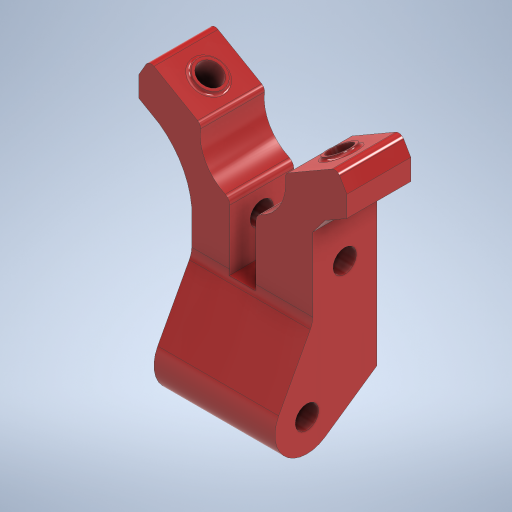
# Autodesk Inventor part: YZ_Roller
Saved by Autodesk Inventor 2023 (Build 270158000, 158)
## iProperties
Created: 2023-11-24
Part Number: YZ_Roller
Material: Generic
Document SubType Name: Modeling
Designer: danie
Density: 1 g/cm^3
Appearance: Default
Author: danie
Autodesk Inventor part; units mm, degrees
ref_plane "YZ Plane" through (0, 0, 0) normal (1, 0, 0) x (0, 1, 0)
ref_plane "XZ Plane" through (0, 0, 0) normal (0, 1, 0) x (-1, 0, 0)
ref_plane "XY Plane" through (0, 0, 0) normal (0, 0, 1) x (1, 0, 0)
sketch "Sketch1" plane through (59.7334, 64.5979, 5.1545) normal (1, 0, 0) x (0, 1, 0)
  line L0 (18.8189, 17.1759) -> (22.8279, 17.1759) projected
  line L1 (18.8189, -4.3241) -> (22.8279, -4.3241) projected
  line L2 (22.3279, -4.8241) -> (19.3338, -4.8241) projected
  arc A0 (-48.3948, 28.867) -> (-62.6447, 12.9256) centre (-53.5949, 19.1757) ccw
  line L3 (-48.3948, 28.867) -> (-28.1429, 18.0072)
  line L4 (-24.8341, 17.1759) -> (22.8279, 17.1759)
  line L5 (22.8279, 17.1759) -> (22.8279, -4.3241)
  line L6 (22.8279, -4.3241) -> (22.8279, -4.8241)
  line L7 (22.8279, -4.8241) -> (22.3279, -4.8241)
  line L8 (22.3279, -4.8241) -> (-50.3885, -4.8241)
  line L9 (-50.3885, -4.8241) -> (-62.6447, 12.9256)
  arc A1 (-28.1429, 18.0072) -> (-24.8341, 17.1759) centre (-24.8333, 24.1792) ccw
  point P0 (-48.3934, 28.8694)
  point P1 (0.4728, 17.1759)
  point P2 (-13.5862, 6.178)
  constraints: 14 end point, 4 point on circle, 2 centre point, 2 perpendicular, 1 coincident, 1 collinear, 1 horizontal, 1 point on line, 1 tangent
sketch "Sketch2" plane through (47.0121, 65.2772, 22.3304) normal (0, 0, 1) x (1, 0, 0)
  line L0 (17.0615, 5.4672) -> (24.4547, 9.7356)
  line L1 (24.4547, 9.7356) -> (24.4547, 16.9356)
  line L2 (24.4547, 16.9356) -> (22.0224, 21.1485)
  arc A0 (22.0224, 21.1485) -> (19.2903, 21.8806) centre (20.2903, 20.1485) ccw
  line L3 (22.0224, 21.1485) -> (20.2903, 20.1485) construction
  line L4 (19.2903, 21.8806) -> (20.2903, 20.1485) construction
  line L5 (19.2903, 21.8806) -> (4.2935, 13.2221)
  arc A1 (4.2935, 13.2221) -> (3.3088, 11.2431) centre (5.2935, 11.4901) ccw
  arc A2 (-25.8662, 11.2431) -> (3.3088, 11.2431) centre (-11.2787, 9.4277) ccw
  arc A3 (-25.8662, 11.2431) -> (-26.8509, 13.2221) centre (-27.8509, 11.4901) ccw
  line L6 (-26.8509, 13.2221) -> (-41.8477, 21.8806)
  arc A4 (-41.8477, 21.8806) -> (-44.5798, 21.1485) centre (-42.8477, 20.1485) ccw
  line L7 (-44.5798, 21.1485) -> (-47.0121, 16.9356)
  line L8 (-47.0121, 16.9356) -> (-47.0121, 16.9356)
  line L9 (-47.0121, 9.7356) -> (-39.9003, 5.6296) projected
  line L10 (-39.926, 5.6445) -> (-39.2899, 5.1683) projected
  line L11 (-39.926, 5.6445) -> (-47.0121, 9.7356)
  arc A5 (-28.8787, -13.5153) -> (-39.926, 5.6445) centre (-55.4557, -16.0746) ccw
  line L12 (12.7213, -0.2066) -> (17.0615, 5.4672)
  line L13 (12.7213, -65.2726) -> (12.7213, -49.0741) projected
  line L14 (12.7213, -65.2726) -> (12.7213, -25.5127)
  line L15 (12.7213, -65.2726) -> (-28.8787, -65.2726)
  line L16 (12.7213, -25.5127) -> (12.7213, -0.2066)
  line L17 (-28.8787, -65.2726) -> (-28.8787, -13.5153)
  line L18 (-47.0121, 9.7356) -> (-47.0121, 16.9356)
  line L19 (-6.7787, -27.2723) -> (-15.7787, -27.2723) projected
  line L20 (-6.7787, -27.2723) -> (-15.7787, -27.2723)
  line L21 (-6.7787, -27.2723) -> (-15.7787, -27.2723)
  line L22 (-15.7787, -27.2723) -> (-15.7787, -3.6713)
  line L23 (-15.7787, -3.6713) -> (-6.7787, -3.6713)
  line L24 (-6.7787, -3.6713) -> (-6.7787, -27.2723)
  arc A6 (-15.7787, -6.4085) -> (-17.3582, -3.9562) centre (-18.4721, -6.4085) ccw
  arc A7 (-5.218, -3.9648) -> (-6.7787, -6.384) centre (-4.1232, -6.384) ccw
  point P0 (-47.0121, -65.2772)
  point P1 (12.7213, -49.0728)
  point P2 (12.7213, -63.3241)
  point P3 (-15.7787, -5.7822)
  dimension "d3" = 2
  dimension "d4" = 90
  dimension "d5" = 2
  dimension "d6" = 26.7
  dimension "d7" = 2
  dimension "d8" = 90
  dimension "d13" = 0
  constraints: 42 end point, 18 point on circle, 8 centre point, 8 tangent, 5 vertical, 3 point on line, 2 collinear, 2 horizontal, 2 parallel, 2 perpendicular
  measures "d3" radius of A0
  measures "d4" angle of L3 L4
  measures "d5" radius of A1
  measures "d6" radius of A5
  measures "d7" radius of A4
  measures "d8" angle of L7 L6
  measures "d13" distance from line of L19.end L22
extrude "Extrusion1" add sketch "Sketch1" along normal mid plane 200
extrude "Extrusion2" cut sketch "Sketch2" along normal mid plane 200 contours L12 L16 L14 L13 L15 L17 A5 L9 L18 L7 A4 L6 A3 A2 A6 L22 L19 L24 A7 A1 L5 A0 L2 L1 L0 keep common part
sketch "Sketch5" plane through (35.7334, 74.705, 22.3304) normal (0, 0, 1) x (1, 0, 0)
  point P0 (-35.7334, -74.705)
sketch "Sketch3" plane through (66.3024, 87.1578, 22.3304) normal (-0.4999998, 0.8660255, 0) x (0.8660255, 0.4999998, 0)
  ellipse E0 centre (-8.9999, 10.9997) end of major axis (-4.913, 11.323) minor radius 4.0997 projected
  point P0 (-100.9985, 22.3304)
  constraints: 1 coincident
sketch "Sketch4" plane through (20.1613, 78.4993, 22.3304) normal (0.5000005, 0.8660251, 0) x (0.8660251, -0.5000005, 0)
  ellipse E0 centre (-8.3172, 10.9997) end of major axis (-5.344, 8.1771) minor radius 4.0996 projected
  point P0 (21.7896, 22.3304)
  constraints: 1 coincident
sketch "Sketch6" plane through (18.1334, 14.2094, 0.3304) normal (-1, 0, 0) x (0, 0, 1)
  point P0 (-0.3304, -14.2094)
hole "Hole1" at (58.5083, 82.6578, 11.3306) direction (0.4999998, -0.8660255, 0) diameter 8 end through all clearance for "Countersunk Flat Head Screw ISO 2009/7046" size "M8" standard "ISO"
hole "Hole2" at (12.9584, 82.6579, 11.3307) direction (-0.5000005, -0.8660251, 0) diameter 8 end through all clearance for "Slotted Cheese Head Screw ISO 1207" size "M8" standard "ISO"
hole "Hole3" at (59.7334, 51.0116, 11.3325) at (59.7334, 11.003, 24.3302) direction (-1, 0, 0) diameter 8 end through all
sketch "Sketch7" plane through (0, 75.0129, 0.3304) normal (-0.4999998, -0.8660255, 0) x (0.8660255, -0.4999998, 0)
  arc A0 (8.1823, 14.923) -> (8.1823, 7.0776) centre (7.3997, 11.0003) ccw projected
  line L0 (8.1823, 14.923) -> (8.1823, 22) projected
  line L1 (8.1823, 22) -> (0, 22) projected
  line L2 (0, 0) -> (0, 22) projected
  line L3 (0, 0) -> (8.1823, 0) projected
  line L4 (8.1823, 0) -> (8.1823, 7.0776) projected
  circle A1 centre (7.3997, 11.0003) radius 7
  point P0 (37.5064, -0.3304)
  dimension "d39" = 14
  constraints: 1 centre point, 1 coincident
  measures "d39" diameter of A1
extrude "Extrusion5" cut sketch "Sketch7" along normal blind 10 contours L0 A1 L4 A0 | A0 L4 A1 L0
sketch "Sketch8" plane through (71.4668, 75.0129, 0.3304) normal (0.5000009, -0.8660249, 0) x (0.8660249, 0.5000009, 0)
  arc A0 (-8.5369, 7.1652) -> (-8.5369, 14.8353) centre (-7.4, 11.0003) ccw projected
  line L0 (-8.5369, 0) -> (-8.5369, 7.1652) projected
  line L1 (-8.5369, 0) -> (0, 0) projected
  line L2 (0, 0) -> (0, 22) projected
  line L3 (0, 22) -> (-8.5369, 22) projected
  line L4 (-8.5369, 14.8353) -> (-8.5369, 22) projected
  circle A1 centre (-7.4, 11.0003) radius 7
  point P0 (-99.3985, -0.3304)
  dimension "d3" = 2
  dimension "d4" = 90
  dimension "d42" = 14
  constraints: 1 centre point, 1 coincident
  measures "d42" diameter of A1
extrude "Extrusion6" cut sketch "Sketch8" along normal blind 10 contours L0 A1 L4 A0 | A0 L4 A1 L0
sketch "Sketch9" plane through (51.3056, 78.4993, 22.3304) normal (-0.4999998, 0.8660255, 0) x (0.8660255, 0.4999998, 0)
  circle A0 centre (8.3169, 10.9997) radius 4 projected
  line L0 (17.3169, 22) -> (0, 22) projected
  line L1 (0, 22) -> (0, 0) projected
  line L2 (0, 0) -> (17.3169, 0) projected
  line L3 (17.3169, 22) -> (17.3169, 0) projected
  circle A1 centre (8.3169, 10.9997) radius 6
  point P0 (-83.6816, 22.3304)
  dimension "d57" = 2
  constraints: 1 centre point
  measures "d57" radial gap between concentric circles of A0 A1
sketch "Sketch10" plane through (5.1644, 87.1578, 22.3304) normal (0.5000005, 0.8660251, 0) x (0.8660251, -0.5000005, 0)
  circle A0 centre (8.9997, 10.9997) radius 4 projected
  line L0 (17.3169, 22) -> (0, 22) projected
  line L1 (0, 22) -> (0, 0) projected
  line L2 (0, 0) -> (17.3169, 0) projected
  line L3 (17.3169, 22) -> (17.3169, 0) projected
  circle A1 centre (8.9997, 10.9997) radius 6
  point P0 (39.1065, 22.3304)
  dimension "d50" = 2
  constraints: 1 centre point
  measures "d50" radial gap between concentric circles of A0 A1
sketch "Sketch11" plane through (40.2334, 38.0049, 0.3304) normal (-1, 0, 0) x (0, 0, 1)
  circle A0 centre (11.0021, 13.0067) radius 4 projected
  line L0 (0, 20.8883) -> (0, 0) projected
  line L1 (0, 0) -> (22.2247, 0) projected
  arc A1 (22, 1.7588) -> (22.2247, 0) centre (29.0033, 1.7597) ccw projected
  line L2 (22, 1.7588) -> (22, 20.8883) projected
  line L3 (0, 20.8883) -> (22, 20.8883) projected
  circle A2 centre (11.0021, 13.0067) radius 6
  point P0 (-0.3304, -38.0049)
  dimension "d54" = 2
  constraints: 1 centre point
  measures "d54" radial gap between concentric circles of A0 A2
extrude "Extrusion10" add sketch "Sketch9" along normal blind 1 contours A1
extrude "Extrusion11" add sketch "Sketch10" along normal blind 1 contours A1
extrude "Extrusion12" add sketch "Sketch11" along normal blind 1 contours A2
fillet "Fillet3" radius 1 3 edges at (52.8121, 80.5238, 11.3306) (39.2334, 51.0116, 5.3325) (8.2622, 86.524, 11.3307) inverted yes
body "Solid1"
